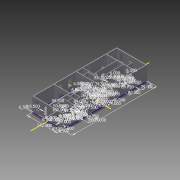
# Autodesk Inventor part: 2nd Floor
Saved by Autodesk Inventor 2013 SP2 (Build 170200200, 200)
## iProperties
Created: 2013-06-25
Part Number: 2nd Floor
Material: Generic
Document SubType Name: Modeling
Designer: Joey
Density: 1 g/cm^3
Author: Joey
Autodesk Inventor part; units mm, degrees
ref_plane "YZ Plane" through (0, 0, 0) normal (1, 0, 0) x (0, 1, 0)
ref_plane "XZ Plane" through (0, 0, 0) normal (0, 1, 0) x (-1, 0, 0)
ref_plane "XY Plane" through (0, 0, 0) normal (0, 0, 1) x (1, 0, 0)
sketch "Sketch1" plane through (0, 0, 0) normal (0, 1, 0) x (-1, 0, 0)
  line L0 (4302.76, 0) -> (-4302.76, 0) projected
  line L1 (0, -12001.5) -> (0, 12001.5) projected
  line L2 (3073.4, -8572.5) -> (-3073.4, -8572.5)
  line L3 (-3073.4, -8572.5) -> (-3073.4, 8572.5)
  line L4 (-3073.4, 8572.5) -> (3073.4, 8572.5)
  line L5 (3073.4, 8572.5) -> (3073.4, -8572.5)
  line L6 (2908.3, -8407.4) -> (-2908.3, -8407.4)
  line L7 (-2908.3, -8407.4) -> (-2908.3, 8407.4)
  line L8 (-2908.3, 5803.9) -> (-2908.3, 5918.2)
  line L9 (-2908.3, 8407.4) -> (-279.4, 8407.4)
  line L10 (-482.6, 8407.4) -> (2908.3, 8407.4)
  line L11 (2908.3, 8407.4) -> (2908.3, 4159.25)
  line L12 (2908.3, 4044.95) -> (2908.3, -8407.4)
  line L13 (-774.7, -292.1) -> (-774.7, -139.7)
  line L14 (2908.3, -139.7) -> (2908.3, -292.1)
  line L15 (961.4159, -292.1) -> (876.3, -292.1)
  line L16 (-514.35, -1485.9) -> (1289.2959, -1485.9)
  line L17 (2908.3, -1485.9) -> (2908.3, -1600.2)
  line L18 (806.45, -1600.2) -> (692.15, -1600.2)
  line L19 (692.15, -6248.4) -> (806.45, -6248.4)
  line L20 (692.15, -6248.4) -> (2908.3, -6248.4)
  line L21 (2908.3, -6248.4) -> (2908.3, -6400.8)
  line L22 (2908.3, -6400.8) -> (692.15, -6400.8)
  line L23 (692.15, -6400.8) -> (692.15, -6248.4)
  line L24 (-279.4, 4876.8) -> (-1993.9, 4876.8)
  line L25 (-2908.3, 4508.5) -> (-2908.3, 4394.2)
  line L26 (-2908.3, 2717.8) -> (-774.7, 2717.8)
  line L27 (-774.7, 2717.8) -> (-774.7, 2832.1)
  line L28 (-774.7, 2832.1) -> (-2908.3, 2832.1)
  line L29 (-2908.3, 2832.1) -> (-2908.3, 2717.8)
  line L30 (-774.7, -292.1) -> (-660.4, -292.1)
  line L31 (-2908.3, -1104.9) -> (-1504.95, -1104.9)
  line L32 (-1504.95, -1104.9) -> (-1504.95, -990.6)
  line L33 (-1504.95, -990.6) -> (-2908.3, -990.6)
  line L34 (-2908.3, -990.6) -> (-2908.3, -1104.9)
  line L35 (-2908.3, -1714.5) -> (-1504.95, -1714.5)
  line L36 (-1504.95, -1714.5) -> (-1504.95, -1600.2)
  line L37 (-1504.95, -1600.2) -> (-2908.3, -1600.2)
  line L38 (-2908.3, -1600.2) -> (-2908.3, -1714.5)
  line L39 (-2908.3, -139.7) -> (-2908.3, -292.1)
  line L40 (-774.7, -292.1) -> (-774.7, -139.7)
  line L41 (-514.35, -2616.2) -> (-514.35, -2730.5)
  line L42 (-2908.3, -2730.5) -> (-2908.3, -2616.2)
  line L43 (-514.35, -2616.2) -> (-628.65, -2616.2)
  line L44 (-628.65, -2616.2) -> (-628.65, -4235.45)
  line L45 (-628.65, -4235.45) -> (-514.35, -4235.45)
  line L46 (-514.35, -4235.45) -> (-514.35, -2616.2)
  line L47 (-514.35, -4235.45) -> (-2908.3, -4235.45)
  line L48 (-2908.3, -4235.45) -> (-2908.3, -4349.75)
  line L49 (-2908.3, -4349.75) -> (-514.35, -4349.75)
  line L50 (-514.35, -4349.75) -> (-514.35, -4235.45)
  line L51 (-514.35, -4349.75) -> (-628.65, -4349.75)
  line L52 (-628.65, -6248.4) -> (-514.35, -6248.4)
  line L53 (-514.35, -6248.4) -> (-2908.3, -6248.4)
  line L54 (-2908.3, -6248.4) -> (-2908.3, -6400.8)
  line L55 (-2908.3, -6400.8) -> (-514.35, -6400.8)
  line L56 (-514.35, -6400.8) -> (-514.35, -6248.4)
  line L57 (1670.05, -1600.2) -> (1555.75, -1600.2)
  line L58 (1555.75, -1600.2) -> (1555.75, -292.1)
  line L59 (1555.75, -292.1) -> (1670.05, -292.1)
  line L60 (1670.05, -292.1) -> (1670.05, -1600.2)
  line L61 (-2813.05, 5918.2) -> (-2908.3, 5918.2)
  line L62 (-2908.3, 8407.4) -> (-2813.05, 8407.4)
  line L63 (-660.4, 4762.5) -> (-774.7, 4762.5)
  line L64 (-774.7, 4762.5) -> (-774.7, 3625.85)
  line L65 (-774.7, 3625.85) -> (-660.4, 3625.85)
  line L66 (-660.4, 3625.85) -> (-660.4, 4762.5)
  line L67 (-514.35, -1485.9) -> (-514.35, -1600.2)
  line L68 (-1504.95, -292.1) -> (-1390.65, -292.1)
  line L69 (-1390.65, -292.1) -> (-1390.65, -2616.2)
  line L70 (-1390.65, -2616.2) -> (-1504.95, -2616.2)
  line L71 (-1504.95, -2616.2) -> (-1504.95, -292.1)
  line L72 (-2070.1, -292.1) -> (-1955.8, -292.1)
  line L73 (-1955.8, -292.1) -> (-1955.8, -1600.2)
  line L74 (-1955.8, -1600.2) -> (-2070.1, -1600.2)
  line L75 (-2070.1, -1600.2) -> (-2070.1, -292.1)
  line L76 (1555.75, -1320.8) -> (-514.35, -1320.8)
  line L77 (-514.35, -1320.8) -> (-514.35, -1206.5)
  line L78 (-514.35, -1206.5) -> (1555.75, -1206.5)
  line L79 (1555.75, -1206.5) -> (1555.75, -1320.8)
  line L80 (-514.35, -1206.5) -> (-400.05, -1206.5)
  line L81 (-400.05, -1206.5) -> (-400.05, -1600.2)
  line L82 (-400.05, -1600.2) -> (-514.35, -1600.2)
  line L83 (-514.35, -1600.2) -> (-514.35, -1206.5)
  line L84 (196.85, -139.7) -> (196.85, -292.1)
  line L85 (876.3, -139.7) -> (876.3, -292.1)
  line L86 (-2527.3, 8407.4) -> (-2413, 8407.4)
  line L87 (-2413, 8407.4) -> (-2413, 5918.2)
  line L88 (-2413, 5918.2) -> (-2527.3, 5918.2)
  line L89 (-2527.3, 5918.2) -> (-2527.3, 8407.4)
  line L90 (-774.7, -139.7) -> (196.85, -139.7)
  line L91 (876.3, -139.7) -> (2908.3, -139.7)
  line L92 (2908.3, -292.1) -> (876.3, -292.1)
  line L93 (196.85, -292.1) -> (-774.7, -292.1)
  line L94 (-514.35, -6248.4) -> (-311.15, -6248.4)
  line L95 (-311.15, -6248.4) -> (-311.15, -6400.8)
  line L96 (-311.15, -6400.8) -> (-514.35, -6400.8)
  line L97 (-514.35, -6400.8) -> (-514.35, -6248.4)
  line L98 (692.15, -6248.4) -> (488.95, -6248.4)
  line L99 (488.95, -6248.4) -> (488.95, -6400.8)
  line L100 (488.95, -6400.8) -> (692.15, -6400.8)
  line L101 (692.15, -6400.8) -> (692.15, -6248.4)
  line L102 (-774.7, -6400.8) -> (-660.4, -6400.8)
  line L103 (-1593.85, 5918.2) -> (-1657.35, 5918.2)
  line L104 (-1993.9, 4762.5) -> (-1879.6, 4762.5)
  line L105 (-660.4, 2832.1) -> (-660.4, 2870.2)
  line L106 (-660.4, 2870.2) -> (-774.7, 2870.2)
  line L107 (-774.7, 2870.2) -> (-774.7, 2832.1)
  line L108 (2908.3, 4159.25) -> (2908.3, 4044.95)
  line L109 (-127, 3956.05) -> (-279.4, 3956.05)
  line L110 (-279.4, 8407.4) -> (-127, 8407.4)
  line L111 (-1993.9, 3841.75) -> (-1993.9, 3956.05)
  line L112 (-1993.9, 5918.2) -> (-1879.6, 5918.2)
  line L113 (-1879.6, 4762.5) -> (-1993.9, 4762.5)
  line L114 (234.95, -1600.2) -> (349.25, -1600.2)
  line L115 (349.25, -1600.2) -> (349.25, -1905)
  line L116 (349.25, -1905) -> (234.95, -1905)
  line L117 (234.95, -1905) -> (234.95, -1600.2)
  line L118 (234.95, -1790.7) -> (692.15, -1790.7)
  line L119 (692.15, -1790.7) -> (692.15, -1905)
  line L120 (692.15, -1905) -> (234.95, -1905)
  line L121 (234.95, -1905) -> (234.95, -1790.7)
  line L122 (-127, 3956.05) -> (-127, 3841.75)
  line L123 (-127, 4191) -> (749.3, 4191)
  line L124 (749.3, 4191) -> (749.3, 4343.4)
  line L125 (749.3, 4343.4) -> (-127, 4343.4)
  line L126 (-127, 4343.4) -> (-127, 4191)
  line L127 (2032, 4191) -> (2908.3, 4191)
  line L128 (2908.3, 4191) -> (2908.3, 4343.4)
  line L129 (2908.3, 4343.4) -> (2032, 4343.4)
  line L130 (2032, 4343.4) -> (2032, 4191)
  line L131 (-1993.9, 3841.75) -> (-1879.6, 3841.75)
  line L132 (-1879.6, 3841.75) -> (-1879.6, 4762.5)
  line L133 (-1879.6, 4762.5) -> (-1993.9, 4762.5)
  line L134 (-1993.9, 4762.5) -> (-1993.9, 3841.75)
  line L135 (-1879.6, 3841.75) -> (-1993.9, 3841.75)
  line L136 (-279.4, 5918.2) -> (-279.4, 5803.9)
  line L137 (-279.4, 4876.8) -> (-279.4, 4762.5)
  line L138 (-1993.9, 4762.5) -> (-1879.6, 4762.5)
  line L139 (-1993.9, 4762.5) -> (-279.4, 4762.5)
  line L140 (-1993.9, 4876.8) -> (-2908.3, 4876.8)
  line L141 (-1993.9, 4762.5) -> (-2908.3, 4762.5)
  line L142 (-1231.9, -6400.8) -> (-1117.6, -6400.8)
  line L143 (-1117.6, -6400.8) -> (-1117.6, -7442.2)
  line L144 (-1117.6, -7442.2) -> (-1231.9, -7442.2)
  line L145 (-1231.9, -7442.2) -> (-1231.9, -6400.8)
  line L146 (692.15, -6045.2) -> (806.45, -6045.2)
  line L147 (692.15, -5334) -> (806.45, -5334)
  line L148 (692.15, -6045.2) -> (692.15, -6248.4)
  line L149 (806.45, -6248.4) -> (806.45, -6045.2)
  line L150 (-628.65, -4425.95) -> (-514.35, -4425.95)
  line L151 (-628.65, -5226.05) -> (-514.35, -5226.05)
  line L152 (692.15, -2971.8) -> (806.45, -2971.8)
  line L153 (692.15, -3771.9) -> (806.45, -3771.9)
  line L154 (692.15, -1600.2) -> (692.15, -2971.8)
  line L155 (692.15, -3771.9) -> (692.15, -5334)
  line L156 (806.45, -5334) -> (806.45, -3771.9)
  line L157 (806.45, -2971.8) -> (806.45, -1600.2)
  line L158 (-1339.85, -2616.2) -> (-1339.85, -2730.5)
  line L159 (-730.25, -2616.2) -> (-730.25, -2730.5)
  line L160 (-1555.75, -2616.2) -> (-1555.75, -2730.5)
  line L161 (-2165.35, -2616.2) -> (-2165.35, -2730.5)
  line L162 (-2165.35, -2730.5) -> (-2908.3, -2730.5)
  line L163 (-2908.3, -2616.2) -> (-2165.35, -2616.2)
  line L164 (-1555.75, -2616.2) -> (-1339.85, -2616.2)
  line L165 (-730.25, -2616.2) -> (-514.35, -2616.2)
  line L166 (-514.35, -2730.5) -> (-730.25, -2730.5)
  line L167 (-1339.85, -2730.5) -> (-1555.75, -2730.5)
  line L168 (-774.7, 1492.25) -> (-660.4, 1492.25)
  line L169 (-774.7, 736.6) -> (-660.4, 736.6)
  line L170 (-660.4, -292.1) -> (-660.4, 736.6)
  line L171 (-660.4, 1492.25) -> (-660.4, 2832.1)
  line L172 (-774.7, 2832.1) -> (-774.7, 1492.25)
  line L173 (-774.7, 736.6) -> (-774.7, -292.1)
  line L174 (-279.4, 8242.3) -> (-127, 8242.3)
  line L175 (-279.4, 7442.2) -> (-127, 7442.2)
  line L176 (-1447.8, 5918.2) -> (-1333.5, 5918.2)
  line L177 (-1333.5, 5918.2) -> (-1333.5, 4762.5)
  line L178 (-1333.5, 4762.5) -> (-1447.8, 4762.5)
  line L179 (-1447.8, 4762.5) -> (-1447.8, 5918.2)
  line L180 (-1993.9, 3956.05) -> (-1631.95, 3956.05)
  line L181 (-1631.95, 3956.05) -> (-1631.95, 3841.75)
  line L182 (-1631.95, 3841.75) -> (-1993.9, 3841.75)
  line L183 (-1993.9, 3841.75) -> (-1993.9, 3956.05)
  line L184 (-127, 3841.75) -> (-1022.35, 3841.75)
  line L185 (-1022.35, 3841.75) -> (-1022.35, 3956.05)
  line L186 (-1022.35, 3956.05) -> (-127, 3956.05)
  line L187 (-127, 3956.05) -> (-127, 3841.75)
  line L188 (-1111.25, 5918.2) -> (-1111.25, 5803.9)
  line L189 (-501.65, 5918.2) -> (-501.65, 5803.9)
  line L190 (-2908.3, 5918.2) -> (-1111.25, 5918.2)
  line L191 (-501.65, 5918.2) -> (-279.4, 5918.2)
  line L192 (-279.4, 5803.9) -> (-501.65, 5803.9)
  line L193 (-1111.25, 5803.9) -> (-2908.3, 5803.9)
  line L194 (-127, 8407.4) -> (-127, 8242.3)
  line L195 (-127, 7442.2) -> (-127, 3956.05)
  line L196 (-279.4, 3956.05) -> (-279.4, 7442.2)
  line L197 (-279.4, 8242.3) -> (-279.4, 8407.4)
  line L198 (-2794, -139.7) -> (-2794, -292.1)
  line L199 (-2184.4, -139.7) -> (-2184.4, -292.1)
  line L200 (-774.7, -139.7) -> (-2184.4, -139.7)
  line L201 (-2794, -139.7) -> (-2908.3, -139.7)
  line L202 (-2908.3, -292.1) -> (-2794, -292.1)
  line L203 (-2184.4, -292.1) -> (-774.7, -292.1)
  line L204 (2806.7, -1485.9) -> (2806.7, -1600.2)
  line L205 (2051.05, -1600.2) -> (2051.05, -1485.9)
  line L206 (-628.65, -4349.75) -> (-628.65, -4425.95)
  line L207 (-628.65, -5226.05) -> (-628.65, -6248.4)
  line L208 (-514.35, -6248.4) -> (-514.35, -5226.05)
  line L209 (-514.35, -4425.95) -> (-514.35, -4349.75)
  line L210 (2908.3, -1600.2) -> (2806.7, -1600.2)
  line L211 (2051.05, -1600.2) -> (-514.35, -1600.2)
  line L212 (-514.35, -1485.9) -> (2051.05, -1485.9)
  line L213 (2806.7, -1485.9) -> (2908.3, -1485.9)
  line L214 (-1993.9, 4876.8) -> (-1993.9, 4762.5)
  line L215 (-1231.9, -7327.9) -> (-520.7, -7327.9)
  line L216 (-520.7, -7327.9) -> (-520.7, -7442.2)
  line L217 (-520.7, -7442.2) -> (-1231.9, -7442.2)
  line L218 (-1231.9, -7442.2) -> (-1231.9, -7327.9)
  line L219 (-774.7, 2870.2) -> (-660.4, 2870.2)
  line L220 (-660.4, 2870.2) -> (-660.4, 1492.25)
  line L221 (-660.4, 1492.25) -> (-774.7, 1492.25)
  line L222 (-774.7, 1492.25) -> (-774.7, 2870.2)
  line L223 (-2908.3, 2832.1) -> (-2908.3, 4762.5)
  line L224 (-2908.3, 4876.8) -> (-2908.3, 5803.9)
  line L225 (-2908.3, 5918.2) -> (-2527.3, 5918.2)
  line L226 (-2908.3, 5918.2) -> (-2908.3, 8407.4)
  line L227 (-2908.3, 8407.4) -> (-279.4, 8407.4)
  line L228 (2908.3, 8407.4) -> (2908.3, 4343.4)
  line L229 (2908.3, 4191) -> (2908.3, -139.7)
  line L230 (-2908.3, 4876.8) -> (-279.4, 4876.8)
  line L231 (-279.4, 4876.8) -> (-279.4, 4762.5)
  line L232 (-279.4, 4762.5) -> (-2908.3, 4762.5)
  line L233 (-2908.3, 4762.5) -> (-2908.3, 4876.8)
  line L234 (-2908.3, 8407.4) -> (2908.3, 8407.4)
  line L235 (2908.3, 8407.4) -> (2908.3, -8407.4)
  line L236 (2908.3, -8407.4) -> (-2908.3, -8407.4)
  line L237 (-2908.3, -8407.4) -> (-2908.3, 8407.4)
  point P0 (0, 0)
  point P1 (-2470.15, 8407.4)
  point P2 (-2908.3, 5861.05)
  point P3 (-2908.3, 2774.95)
  point P4 (-2908.3, -215.9)
  point P5 (-2908.3, -1047.75)
  point P6 (-2908.3, -1657.35)
  point P7 (-2908.3, -2673.35)
  point P8 (-2908.3, -4292.6)
  point P9 (-2908.3, -6324.6)
  point P10 (2908.3, -1543.05)
  point P11 (2908.3, -6324.6)
  point P12 (2908.3, -215.9)
  point P13 (-203.2, 8407.4)
  dimension "d0" = 17145
  dimension "d2" = 6146.8
  dimension "d14" = 165.1
  dimension "d15" = 165.1
  dimension "d22" = 152.4
  dimension "d25" = 114.3
  dimension "d30" = 114.3
  dimension "d36" = 114.3
  dimension "d38" = 114.3
  dimension "d42" = 152.4
  dimension "d44" = 114.3
  dimension "d45" = 165.1
  dimension "d54" = 114.3
  dimension "d64" = 165.1
  dimension "d66" = 165.1
  dimension "d67" = 2133.6
  dimension "d71" = 114.3
  dimension "d73" = 2946.4
  dimension "d74" = 114.3
  dimension "d80" = 876.3
  dimension "d81" = 1587.5
  dimension "d82" = 679.45
  dimension "d83" = 114.3
  dimension "d92" = 2032
  dimension "d93" = 152.4
  dimension "d95" = 914.4
  dimension "d96" = 152.4
  dimension "d99" = 203.2
  dimension "d100" = 203.2
  dimension "d112" = 38.1
  dimension "d113" = 755.65
  dimension "d117" = 838.2
  dimension "d128" = 914.4
  dimension "d133" = 114.3
  dimension "d134" = 114.3
  dimension "d137" = 152.4
  dimension "d138" = 1282.7
  dimension "d141" = 114.3
  dimension "d145" = 4064
  dimension "d146" = 876.3
  dimension "d147" = 1009.65
  dimension "d152" = 114.3
  dimension "d162" = 114.3
  dimension "d163" = 114.3
  dimension "d164" = 114.3
  dimension "d165" = 1930.4
  dimension "d166" = 2006.6
  dimension "d173" = 165.1
  dimension "d175" = 1016
  dimension "d176" = 609.6
  dimension "d177" = 114.3
  dimension "d178" = 1041.4
  dimension "d179" = 1676.4
  dimension "d180" = 203.2
  dimension "d181" = 711.2
  dimension "d184" = 114.3
  dimension "d187" = 76.2
  dimension "d188" = 800.1
  dimension "d189" = 2032
  dimension "d191" = 1066.8
  dimension "d192" = 800.1
  dimension "d193" = 1206.5
  dimension "d194" = 2101.85
  dimension "d195" = 457.2
  constraints: 470 end point, 126 parallel, 91 perpendicular, 54 horizontal, 47 collinear, 30 point on line, 13 midpoint, 4 vertical, 16 other
  measures "d0" distance between parallel lines of L4 L2
  measures "d2" distance between parallel lines of L3 L5
  measures "d14" distance between parallel lines of L4 L10
  measures "d15" distance between parallel lines of L4 L9
  measures "d22" distance between parallel lines of L20 L22
  measures "d25" distance between parallel lines of L28 L26
  measures "d30" distance between parallel lines of L37 L35
  measures "d36" distance between parallel lines of L46 L44
  measures "d38" distance between parallel lines of L47 L49
  measures "d42" distance between parallel lines of L53 L55
  measures "d44" distance between parallel lines of L60 L58
  measures "d45" distance between parallel lines of L5 L12
  measures "d54" distance between parallel lines of L66 L64
  measures "d64" distance between parallel lines of L5 L11
  measures "d66" distance between parallel lines of L2 L6
  measures "d71" distance between parallel lines of L75 L73
  measures "d73" distance between parallel lines of L58 L69
  measures "d74" distance between parallel lines of L76 L78
  measures "d80" distance between parallel lines of L69 L83
  measures "d81" distance between parallel lines of L69 L84
  measures "d82" distance between parallel lines of L84 L85
  measures "d83" distance between parallel lines of L89 L87
  measures "d92" distance between parallel lines of L12 L85
  measures "d93" distance between parallel lines of L92 L91
  measures "d95" distance between parallel lines of L78 L93
  measures "d96" distance between parallel lines of L93 L90
  measures "d99" distance between parallel lines of L97 L95
  measures "d100" distance between parallel lines of L101 L99
  measures "d112" distance between parallel lines of L28 L106
  measures "d113" distance between parallel lines of L106 L65
  measures "d133" distance between parallel lines of L120 L118
  measures "d134" distance between parallel lines of L117 L115
  measures "d137" distance between parallel lines of L123 L125
  measures "d138" distance between parallel lines of L130 L124
  measures "d141" distance between parallel lines of L134 L132
  measures "d145" distance between parallel lines of L129 L10
  measures "d146" distance from line of L12.start L130
  measures "d147" distance between parallel lines of L28 L131
  measures "d152" distance between parallel lines of L139 L24
  measures "d162" distance between parallel lines of L83 L81
  measures "d163" distance between parallel lines of L31 L33
  measures "d164" distance between parallel lines of L69 L71
  measures "d165" distance between parallel lines of L28 L139
  measures "d166" distance between parallel lines of L6 L55
  measures "d175" distance of point (-2908.3, -2673.35) point (-2908.3, -1657.35)
  measures "d176" distance of point (-2908.3, -1047.75) point (-2908.3, -1657.35)
  measures "d177" distance between parallel lines of L145 L143
  measures "d178" distance between parallel lines of L102 L144
  measures "d180" distance between parallel lines of L98 L146
  measures "d181" distance between parallel lines of L146 L147
  measures "d184" distance between parallel lines of L149 L148
  measures "d187" distance between parallel lines of L49 L150
  measures "d188" distance between parallel lines of L151 L150
  measures "d189" distance of point (-2908.3, -6324.6) point (-2908.3, -4292.6)
  measures "d191" distance between parallel lines of L120 L152
  measures "d192" distance between parallel lines of L152 L153
  measures "d193" distance between parallel lines of L46 L155
  measures "d194" distance between parallel lines of L12 L156
  measures "d195" distance between parallel lines of L154 L117
extrude "Extrusion1" add sketch "Sketch1" along normal blind 2844.8 contours L5 L2 L1 L6 L12 L0 | L0 L12 L108 L11 L10 L1 L4 L5 | L12 L92 L59 L15 L85 L91 | L1 L10 L9 L7 L0 L3 L4 | L2 L3 L0 L7 L6 L1 | L170 L90 L173 L0 | L0 L173 L169 L170 | L90 L84 L93 L1 | L1 L93 L170 L90 | L123 L126 L125 L1 | L1 L125 L124 L123 | L170 L30 L13 L90 | L195 L109 L196 L137 L136 L175 L126 | L127 L130 L129 L11 | L12 L210 L204 L213 | L60 L212 L58 L59 | L194 L174 L197 L10 | L211 L81 L16 L1 | L1 L16 L212 L58 L211 L18 L114 | L13 L203 L68 L72 L199 L200 | L78 L58 L76 L1 | L1 L76 L81 L78 | L122 L184 L66 L186 L109 | L212 L205 L211 L60 | L60 L57 L58 L212 | L114 L115 L118 L117 | L82 L67 L16 L81 | L22 L23 L19 L20 L12 | L7 L53 L52 L56 L55 | L201 L198 L202 L7 | L7 L28 L27 L26 | L81 L76 L77 L78 | L16 L83 L76 L81 | L211 L154 L118 L115 | L118 L115 L116 L117 | L100 L99 L98 L23 | L55 L143 L215 L145 | L27 L107 L106 L105 L171 L168 L172 | L69 L70 L71 L36 L32 L68 | L186 L64 L63 L66 | L66 L184 L64 L186 | L139 L63 L177 L24 L137 | L66 L65 L64 L184 | L19 L148 L146 L149 | L87 L88 L89 L9 | L118 L119 L120 L115 | L18 L157 L152 L154 L119 | L7 L47 L45 L50 L49 | L207 L151 L208 L52 | L215 L143 L144 L145 | L33 L75 L31 L7 | L164 L158 L167 L160 L70 | L72 L73 L33 L75 | L136 L192 L189 L191 | L64 L184 L185 L186 | L190 L112 L103 L179 L193 L7 L61 L88 | L49 L209 L150 L206 | L94 L95 L96 L56 | L215 L216 L217 L143 | L33 L73 L31 L75 | L32 L31 L73 L33 | L177 L139 L179 L24 | L24 L179 L193 L177 | L7 L163 L161 L162 | L44 L166 L46 L45 | L37 L36 L35 L7 | L31 L73 L37 L75 | L7 L140 L214 L141 | L179 L139 L104 L214 L24 | L193 L179 L176 L177 | L177 L190 L188 L193 | L166 L159 L165 L44 | L44 L43 L41 L166 | L104 L132 L180 L134 | L180 L132 L131 L111 | L180 L181 L182 L132 | L155 L153 L156 L147
extrude "Extrusion2" add sketch "Sketch1" along normal blind 2844.8 contours L118 L115 L116 L117 | L118 L119 L120 L115
extrude "Extrusion3" cut sketch "Sketch1" along normal blind 2844.8 contours L211 L154 L118 L115
sketch "Sketch2" plane through (0, 0, 0) normal (0, -1, 0) x (1, 0, 0)
  line L0 (1993.9, 3841.75) -> (1631.95, 3841.75) projected
  line L1 (1993.9, 4762.5) -> (1993.9, 3841.75) projected
  line L2 (1231.9, -7442.2) -> (520.7, -7442.2) projected
  line L3 (1231.9, -6400.8) -> (1231.9, -7442.2) projected
  line L4 (-3073.4, 8572.5) -> (3073.4, 8572.5)
  line L5 (3073.4, 8572.5) -> (3073.4, -8572.5)
  line L6 (3073.4, -8572.5) -> (-3073.4, -8572.5)
  line L7 (-3073.4, -8572.5) -> (-3073.4, 8572.5)
  line L8 (520.7, -7442.2) -> (2908.3, -7442.2)
  line L9 (2908.3, -7442.2) -> (2908.3, -8407.4)
  line L10 (2908.3, -8407.4) -> (520.7, -8407.4)
  line L11 (520.7, -8407.4) -> (520.7, -7442.2)
  line L12 (2908.3, -8407.4) -> (1231.9, -8407.4)
  line L13 (1231.9, -8407.4) -> (1231.9, -6400.8)
  line L14 (1231.9, -6400.8) -> (2908.3, -6400.8)
  line L15 (2908.3, -6400.8) -> (2908.3, -8407.4)
  line L16 (1739.9, 3841.75) -> (2908.3, 3841.75)
  line L17 (2908.3, 3841.75) -> (2908.3, 2832.1)
  line L18 (2908.3, 2832.1) -> (1739.9, 2832.1)
  line L19 (1739.9, 2832.1) -> (1739.9, 3841.75)
  line L20 (1993.9, 4762.5) -> (2908.3, 4762.5)
  line L21 (2908.3, 4762.5) -> (2908.3, 2832.1)
  line L22 (2908.3, 2832.1) -> (1993.9, 2832.1)
  line L23 (1993.9, 2832.1) -> (1993.9, 4762.5)
  point P0 (0, 0)
  dimension "d242" = 1168.4
  constraints: 40 end point, 10 parallel, 5 horizontal, 5 perpendicular, 1 point on line
  measures "d242" distance between parallel lines of L17 L19
extrude "Extrusion4" add sketch "Sketch2" along normal blind 463.55
sketch "Sketch3" plane through (0, 2844.8, 0) normal (0, 1, 0) x (1, 0, 0)
  line L0 (-692.15, 1790.7) -> (-349.25, 1790.7) projected
  line L1 (-349.25, 1790.7) -> (-349.25, 1600.2) projected
  line L2 (-349.25, 1600.2) -> (-692.15, 1600.2) projected
  line L3 (-692.15, 1600.2) -> (-692.15, 1790.7) projected
  line L4 (-876.3, 139.7) -> (-2908.3, 139.7) projected
  line L5 (-876.3, 292.1) -> (-876.3, 139.7) projected
  line L6 (-1555.75, 292.1) -> (-876.3, 292.1) projected
  line L7 (-1555.75, 1206.5) -> (-1555.75, 292.1) projected
  line L8 (514.35, 1206.5) -> (-1555.75, 1206.5) projected
  line L9 (514.35, 1600.2) -> (514.35, 1206.5) projected
  line L10 (-234.95, 1600.2) -> (514.35, 1600.2) projected
  line L11 (-234.95, 1600.2) -> (-234.95, 1905) projected
  line L12 (-234.95, 1905) -> (-692.15, 1905) projected
  line L13 (-692.15, 2971.8) -> (-692.15, 1905) projected
  line L14 (-806.45, 6248.4) -> (-2908.3, 6248.4) projected
  line L15 (1390.65, 292.1) -> (1390.65, 2616.2) projected
  line L16 (400.05, 1320.8) -> (400.05, 1485.9) projected
  line L17 (-1555.75, 1320.8) -> (400.05, 1320.8) projected
  line L18 (-1555.75, 1485.9) -> (-1555.75, 1320.8) projected
  line L19 (400.05, 1485.9) -> (-1555.75, 1485.9) projected
  line L20 (-692.15, 5334) -> (-692.15, 3771.9) projected
  line L21 (-806.45, 5334) -> (-692.15, 5334) projected
  line L22 (-806.45, 3771.9) -> (-806.45, 5334) projected
  line L23 (-692.15, 3771.9) -> (-806.45, 3771.9) projected
  line L24 (-1555.75, 292.1) -> (1390.65, 292.1)
  line L25 (1390.65, 292.1) -> (1390.65, 1600.2)
  line L26 (1390.65, 1600.2) -> (-1555.75, 1600.2)
  line L27 (-1555.75, 1600.2) -> (-1555.75, 292.1)
  line L28 (1390.65, 1600.2) -> (-692.15, 1600.2)
  line L29 (-692.15, 1600.2) -> (-692.15, 2616.2)
  line L30 (-692.15, 2616.2) -> (1390.65, 2616.2)
  line L31 (1390.65, 2616.2) -> (1390.65, 1600.2)
  line L32 (-692.15, 2616.2) -> (514.35, 2616.2)
  line L33 (514.35, 2616.2) -> (514.35, 6248.4)
  line L34 (514.35, 6248.4) -> (-692.15, 6248.4)
  line L35 (-692.15, 6248.4) -> (-692.15, 2616.2)
  line L36 (660.4, -4762.5) -> (-2908.3, -4762.5)
  line L37 (-2908.3, -4762.5) -> (-2908.3, 292.1)
  line L38 (-2908.3, 292.1) -> (660.4, 292.1)
  line L39 (660.4, 292.1) -> (660.4, -4762.5)
  line L40 (-2908.3, 292.1) -> (-1555.75, 292.1)
  line L41 (-1555.75, 292.1) -> (-1555.75, 6248.4)
  line L42 (-1555.75, 6248.4) -> (-2908.3, 6248.4)
  line L43 (-2908.3, 6248.4) -> (-2908.3, 292.1)
  line L44 (-692.15, 1600.2) -> (-1555.75, 1600.2)
  line L45 (-1555.75, 1600.2) -> (-1555.75, 6248.4)
  line L46 (-1555.75, 6248.4) -> (-692.15, 6248.4)
  line L47 (-692.15, 6248.4) -> (-692.15, 1600.2)
  line L48 (514.35, 2616.2) -> (2908.3, 2616.2)
  line L49 (2908.3, 2616.2) -> (2908.3, 8407.4)
  line L50 (2908.3, 8407.4) -> (514.35, 8407.4)
  line L51 (514.35, 8407.4) -> (514.35, 2616.2)
  line L52 (2908.3, 8407.4) -> (-2908.3, 8407.4)
  line L53 (-2908.3, 8407.4) -> (-2908.3, 6248.4)
  line L54 (-2908.3, 6248.4) -> (2908.3, 6248.4)
  line L55 (2908.3, 6248.4) -> (2908.3, 8407.4)
  line L56 (-2908.3, -8407.4) -> (2908.3, -8407.4)
  line L57 (2908.3, -8407.4) -> (2908.3, -4762.5)
  line L58 (2908.3, -4762.5) -> (-2908.3, -4762.5)
  line L59 (-2908.3, -4762.5) -> (-2908.3, -8407.4)
  line L60 (-2908.3, -4191) -> (-2603.5, -4191)
  line L61 (-2603.5, -4191) -> (-2603.5, 139.7)
  line L62 (-2603.5, 139.7) -> (-2908.3, 139.7)
  line L63 (-2908.3, 139.7) -> (-2908.3, -4191)
  line L64 (-2908.3, -4762.5) -> (660.4, -4762.5)
  line L65 (660.4, -4762.5) -> (660.4, -4191)
  line L66 (660.4, -4191) -> (-2908.3, -4191)
  line L67 (-2908.3, -4191) -> (-2908.3, -4762.5)
  line L68 (660.4, -4191) -> (-2603.5, -4191)
  line L69 (-2603.5, -4191) -> (-2603.5, 0)
  line L70 (-2603.5, 0) -> (660.4, 0)
  line L71 (660.4, 0) -> (660.4, -4191)
  line L72 (774.7, -2717.8) -> (2908.3, -2717.8) projected
  line L73 (774.7, -2717.8) -> (2908.3, -2717.8)
  line L74 (2908.3, -2717.8) -> (2908.3, 292.1)
  line L75 (2908.3, 292.1) -> (774.7, 292.1)
  line L76 (774.7, 292.1) -> (774.7, -2717.8)
  line L77 (2908.3, 292.1) -> (1390.65, 292.1)
  line L78 (1390.65, 292.1) -> (1390.65, 2616.2)
  line L79 (1390.65, 2616.2) -> (2908.3, 2616.2)
  line L80 (2908.3, 2616.2) -> (2908.3, 292.1)
  line L81 (-692.15, 5334) -> (-806.45, 5334) projected
  line L82 (-692.15, 3771.9) -> (-692.15, 5334) projected
  line L83 (-806.45, 3771.9) -> (-692.15, 3771.9) projected
  line L84 (-806.45, 5334) -> (-806.45, 3771.9) projected
  line L85 (520.7, 7442.2) -> (520.7, 7327.9) projected
  line L86 (520.7, 7442.2) -> (520.7, 8407.4) projected
  line L87 (520.7, 8407.4) -> (-2908.3, 8407.4) projected
  line L88 (-2908.3, 8407.4) -> (-2908.3, 6400.8) projected
  line L89 (-488.95, 6400.8) -> (-2908.3, 6400.8) projected
  line L90 (-488.95, 6248.4) -> (-488.95, 6400.8) projected
  line L91 (-692.15, 6248.4) -> (-488.95, 6248.4) projected
  line L92 (-692.15, 6045.2) -> (-692.15, 6248.4) projected
  line L93 (-806.45, 6045.2) -> (-692.15, 6045.2) projected
  line L94 (-806.45, 6248.4) -> (-806.45, 6045.2) projected
  line L95 (-2908.3, 6248.4) -> (-806.45, 6248.4) projected
  line L96 (-2908.3, 6248.4) -> (-2908.3, 1600.2) projected
  line L97 (-2806.7, 1600.2) -> (-2908.3, 1600.2) projected
  line L98 (-2806.7, 1485.9) -> (-2806.7, 1600.2) projected
  line L99 (-2908.3, 1485.9) -> (-2806.7, 1485.9) projected
  line L100 (-2908.3, 1485.9) -> (-2908.3, 292.1) projected
  line L101 (-1670.05, 292.1) -> (-2908.3, 292.1) projected
  line L102 (-1670.05, 1485.9) -> (-1670.05, 292.1) projected
  line L103 (-2051.05, 1485.9) -> (-1670.05, 1485.9) projected
  line L104 (-2051.05, 1600.2) -> (-2051.05, 1485.9) projected
  line L105 (-806.45, 1600.2) -> (-2051.05, 1600.2) projected
  line L106 (-806.45, 2971.8) -> (-806.45, 1600.2) projected
  line L107 (-692.15, 2971.8) -> (-806.45, 2971.8) projected
  line L108 (-692.15, 1905) -> (-692.15, 2971.8) projected
  line L109 (-234.95, 1905) -> (-692.15, 1905) projected
  line L110 (-234.95, 1600.2) -> (-234.95, 1905) projected
  line L111 (514.35, 1600.2) -> (-234.95, 1600.2) projected
  line L112 (514.35, 1206.5) -> (514.35, 1600.2) projected
  line L113 (-1555.75, 1206.5) -> (514.35, 1206.5) projected
  line L114 (-1555.75, 292.1) -> (-1555.75, 1206.5) projected
  line L115 (-876.3, 292.1) -> (-1555.75, 292.1) projected
  line L116 (-876.3, 139.7) -> (-876.3, 292.1) projected
  line L117 (-2908.3, 139.7) -> (-876.3, 139.7) projected
  line L118 (-2908.3, 139.7) -> (-2908.3, -4191) projected
  line L119 (-2032, -4191) -> (-2908.3, -4191) projected
  line L120 (-2032, -4343.4) -> (-2032, -4191) projected
  line L121 (-2908.3, -4343.4) -> (-2032, -4343.4) projected
  line L122 (-2908.3, -4343.4) -> (-2908.3, -8407.4) projected
  line L123 (-2908.3, -8407.4) -> (127, -8407.4) projected
  line L124 (127, -8242.3) -> (127, -8407.4) projected
  line L125 (279.4, -8242.3) -> (127, -8242.3) projected
  line L126 (279.4, -8407.4) -> (279.4, -8242.3) projected
  line L127 (279.4, -8407.4) -> (2413, -8407.4) projected
  line L128 (2413, -5918.2) -> (2413, -8407.4) projected
  line L129 (1111.25, -5918.2) -> (2413, -5918.2) projected
  line L130 (1111.25, -5803.9) -> (1111.25, -5918.2) projected
  line L131 (1333.5, -5803.9) -> (1111.25, -5803.9) projected
  line L132 (1333.5, -4876.8) -> (1333.5, -5803.9) projected
  line L133 (279.4, -4876.8) -> (1333.5, -4876.8) projected
  line L134 (279.4, -5803.9) -> (279.4, -4876.8) projected
  line L135 (501.65, -5803.9) -> (279.4, -5803.9) projected
  line L136 (501.65, -5918.2) -> (501.65, -5803.9) projected
  line L137 (279.4, -5918.2) -> (501.65, -5918.2) projected
  line L138 (279.4, -7442.2) -> (279.4, -5918.2) projected
  line L139 (127, -7442.2) -> (279.4, -7442.2) projected
  line L140 (127, -4343.4) -> (127, -7442.2) projected
  line L141 (-749.3, -4343.4) -> (127, -4343.4) projected
  line L142 (-749.3, -4191) -> (-749.3, -4343.4) projected
  line L143 (127, -4191) -> (-749.3, -4191) projected
  line L144 (127, -3841.75) -> (127, -4191) projected
  line L145 (660.4, -3841.75) -> (127, -3841.75) projected
  line L146 (660.4, -3625.85) -> (660.4, -3841.75) projected
  line L147 (774.7, -3625.85) -> (660.4, -3625.85) projected
  line L148 (774.7, -3841.75) -> (774.7, -3625.85) projected
  line L149 (1022.35, -3841.75) -> (774.7, -3841.75) projected
  line L150 (1022.35, -3956.05) -> (1022.35, -3841.75) projected
  line L151 (774.7, -3956.05) -> (1022.35, -3956.05) projected
  line L152 (774.7, -4762.5) -> (774.7, -3956.05) projected
  line L153 (1879.6, -4762.5) -> (774.7, -4762.5) projected
  line L154 (1879.6, -3956.05) -> (1879.6, -4762.5) projected
  line L155 (1631.95, -3956.05) -> (1879.6, -3956.05) projected
  line L156 (1631.95, -3841.75) -> (1631.95, -3956.05) projected
  line L157 (1739.9, -3841.75) -> (1631.95, -3841.75) projected
  line L158 (1739.9, -3841.75) -> (1739.9, -2832.1) projected
  line L159 (774.7, -2832.1) -> (1739.9, -2832.1) projected
  line L160 (774.7, -2870.2) -> (774.7, -2832.1) projected
  line L161 (660.4, -2870.2) -> (774.7, -2870.2) projected
  line L162 (660.4, -1492.25) -> (660.4, -2870.2) projected
  line L163 (774.7, -1492.25) -> (660.4, -1492.25) projected
  line L164 (774.7, -2717.8) -> (774.7, -1492.25) projected
  line L165 (2908.3, -2717.8) -> (774.7, -2717.8) projected
  line L166 (2908.3, -2717.8) -> (2908.3, 139.7) projected
  line L167 (2794, 139.7) -> (2908.3, 139.7) projected
  line L168 (2794, 292.1) -> (2794, 139.7) projected
  line L169 (2908.3, 292.1) -> (2794, 292.1) projected
  line L170 (2908.3, 292.1) -> (2908.3, 990.6) projected
  line L171 (2070.1, 990.6) -> (2908.3, 990.6) projected
  line L172 (2070.1, 292.1) -> (2070.1, 990.6) projected
  line L173 (2184.4, 292.1) -> (2070.1, 292.1) projected
  line L174 (2184.4, 139.7) -> (2184.4, 292.1) projected
  line L175 (774.7, 139.7) -> (2184.4, 139.7) projected
  line L176 (774.7, -736.6) -> (774.7, 139.7) projected
  line L177 (660.4, -736.6) -> (774.7, -736.6) projected
  line L178 (660.4, 139.7) -> (660.4, -736.6) projected
  line L179 (-196.85, 139.7) -> (660.4, 139.7) projected
  line L180 (-196.85, 292.1) -> (-196.85, 139.7) projected
  line L181 (1390.65, 292.1) -> (-196.85, 292.1) projected
  line L182 (1390.65, 2616.2) -> (1390.65, 292.1) projected
  line L183 (1339.85, 2616.2) -> (1390.65, 2616.2) projected
  line L184 (1339.85, 2730.5) -> (1339.85, 2616.2) projected
  line L185 (1555.75, 2730.5) -> (1339.85, 2730.5) projected
  line L186 (1555.75, 2616.2) -> (1555.75, 2730.5) projected
  line L187 (1504.95, 2616.2) -> (1555.75, 2616.2) projected
  line L188 (1504.95, 1714.5) -> (1504.95, 2616.2) projected
  line L189 (2908.3, 1714.5) -> (1504.95, 1714.5) projected
  line L190 (2908.3, 1714.5) -> (2908.3, 2616.2) projected
  line L191 (2165.35, 2616.2) -> (2908.3, 2616.2) projected
  line L192 (2165.35, 2730.5) -> (2165.35, 2616.2) projected
  line L193 (2908.3, 2730.5) -> (2165.35, 2730.5) projected
  line L194 (2908.3, 2730.5) -> (2908.3, 4235.45) projected
  line L195 (628.65, 4235.45) -> (2908.3, 4235.45) projected
  line L196 (628.65, 2730.5) -> (628.65, 4235.45) projected
  line L197 (730.25, 2730.5) -> (628.65, 2730.5) projected
  line L198 (730.25, 2616.2) -> (730.25, 2730.5) projected
  line L199 (514.35, 2616.2) -> (730.25, 2616.2) projected
  line L200 (514.35, 4425.95) -> (514.35, 2616.2) projected
  line L201 (628.65, 4425.95) -> (514.35, 4425.95) projected
  line L202 (628.65, 4349.75) -> (628.65, 4425.95) projected
  line L203 (2908.3, 4349.75) -> (628.65, 4349.75) projected
  line L204 (2908.3, 4349.75) -> (2908.3, 6248.4) projected
  line L205 (628.65, 6248.4) -> (2908.3, 6248.4) projected
  line L206 (628.65, 5226.05) -> (628.65, 6248.4) projected
  line L207 (514.35, 5226.05) -> (628.65, 5226.05) projected
  line L208 (514.35, 6248.4) -> (514.35, 5226.05) projected
  line L209 (311.15, 6248.4) -> (514.35, 6248.4) projected
  line L210 (311.15, 6400.8) -> (311.15, 6248.4) projected
  line L211 (1117.6, 6400.8) -> (311.15, 6400.8) projected
  line L212 (1117.6, 7327.9) -> (1117.6, 6400.8) projected
  line L213 (520.7, 7327.9) -> (1117.6, 7327.9) projected
  line L214 (774.7, -3956.05) -> (1879.6, -3956.05)
  line L215 (1879.6, -3956.05) -> (1879.6, -4762.5)
  line L216 (1879.6, -4762.5) -> (774.7, -4762.5)
  line L217 (774.7, -4762.5) -> (774.7, -3956.05)
  line L218 (-488.95, 6400.8) -> (311.15, 6400.8)
  line L219 (311.15, 6400.8) -> (311.15, 6248.4)
  line L220 (311.15, 6248.4) -> (-488.95, 6248.4)
  line L221 (-488.95, 6248.4) -> (-488.95, 6400.8)
  line L222 (-806.45, 6045.2) -> (-692.15, 6045.2)
  line L223 (-692.15, 6045.2) -> (-692.15, 5334)
  line L224 (-692.15, 5334) -> (-806.45, 5334)
  line L225 (-806.45, 5334) -> (-806.45, 6045.2)
  line L226 (514.35, 5226.05) -> (628.65, 5226.05)
  line L227 (628.65, 5226.05) -> (628.65, 4425.95)
  line L228 (628.65, 4425.95) -> (514.35, 4425.95)
  line L229 (514.35, 4425.95) -> (514.35, 5226.05)
  line L230 (-806.45, 3771.9) -> (-692.15, 3771.9)
  line L231 (-692.15, 3771.9) -> (-692.15, 2971.8)
  line L232 (-692.15, 2971.8) -> (-806.45, 2971.8)
  line L233 (-806.45, 2971.8) -> (-806.45, 3771.9)
  line L234 (730.25, 2730.5) -> (1339.85, 2730.5)
  line L235 (1339.85, 2730.5) -> (1339.85, 2616.2)
  line L236 (1339.85, 2616.2) -> (730.25, 2616.2)
  line L237 (730.25, 2616.2) -> (730.25, 2730.5)
  line L238 (1555.75, 2730.5) -> (2165.35, 2730.5)
  line L239 (2165.35, 2730.5) -> (2165.35, 2616.2)
  line L240 (2165.35, 2616.2) -> (1555.75, 2616.2)
  line L241 (1555.75, 2616.2) -> (1555.75, 2730.5)
  line L242 (2184.4, 292.1) -> (2794, 292.1)
  line L243 (2794, 292.1) -> (2794, 139.7)
  line L244 (2794, 139.7) -> (2184.4, 139.7)
  line L245 (2184.4, 139.7) -> (2184.4, 292.1)
  line L246 (1504.95, 990.6) -> (1955.8, 990.6) projected
  line L247 (1504.95, 292.1) -> (1504.95, 990.6) projected
  line L248 (1955.8, 292.1) -> (1504.95, 292.1) projected
  line L249 (1955.8, 990.6) -> (1955.8, 292.1) projected
  line L250 (1955.8, 1104.9) -> (1504.95, 1104.9) projected
  line L251 (1955.8, 1600.2) -> (1955.8, 1104.9) projected
  line L252 (1504.95, 1600.2) -> (1955.8, 1600.2) projected
  line L253 (1504.95, 1104.9) -> (1504.95, 1600.2) projected
  line L254 (2908.3, 1104.9) -> (2070.1, 1104.9) projected
  line L255 (2908.3, 1104.9) -> (2908.3, 1600.2) projected
  line L256 (2070.1, 1600.2) -> (2908.3, 1600.2) projected
  line L257 (2070.1, 1104.9) -> (2070.1, 1600.2) projected
  line L258 (660.4, -736.6) -> (774.7, -736.6)
  line L259 (774.7, -736.6) -> (774.7, -1492.25)
  line L260 (774.7, -1492.25) -> (660.4, -1492.25)
  line L261 (660.4, -1492.25) -> (660.4, -736.6)
  line L262 (660.4, -2870.2) -> (774.7, -2870.2)
  line L263 (774.7, -2870.2) -> (774.7, -3625.85)
  line L264 (774.7, -3625.85) -> (660.4, -3625.85)
  line L265 (660.4, -3625.85) -> (660.4, -2870.2)
  line L266 (1022.35, -3841.75) -> (1631.95, -3841.75)
  line L267 (1631.95, -3841.75) -> (1631.95, -3956.05)
  line L268 (1631.95, -3956.05) -> (1022.35, -3956.05)
  line L269 (1022.35, -3956.05) -> (1022.35, -3841.75)
  line L270 (-2032, -4191) -> (-749.3, -4191)
  line L271 (-749.3, -4191) -> (-749.3, -4343.4)
  line L272 (-749.3, -4343.4) -> (-2032, -4343.4)
  line L273 (-2032, -4343.4) -> (-2032, -4191)
  line L274 (-876.3, 139.7) -> (-196.85, 139.7)
  line L275 (-196.85, 139.7) -> (-196.85, 292.1)
  line L276 (-196.85, 292.1) -> (-876.3, 292.1)
  line L277 (-876.3, 292.1) -> (-876.3, 139.7)
  line L278 (514.35, 1206.5) -> (1390.65, 1206.5)
  line L279 (1390.65, 1206.5) -> (1390.65, 1358.9)
  line L280 (1390.65, 1358.9) -> (514.35, 1358.9)
  line L281 (514.35, 1358.9) -> (514.35, 1206.5)
  line L282 (-2806.7, 1600.2) -> (-2051.05, 1600.2)
  line L283 (-2051.05, 1600.2) -> (-2051.05, 1485.9)
  line L284 (-2051.05, 1485.9) -> (-2806.7, 1485.9)
  line L285 (-2806.7, 1485.9) -> (-2806.7, 1600.2)
  line L286 (501.65, -5803.9) -> (1111.25, -5803.9)
  line L287 (1111.25, -5803.9) -> (1111.25, -5918.2)
  line L288 (1111.25, -5918.2) -> (501.65, -5918.2)
  line L289 (501.65, -5918.2) -> (501.65, -5803.9)
  line L290 (127, -7442.2) -> (279.4, -7442.2)
  line L291 (279.4, -7442.2) -> (279.4, -8242.3)
  line L292 (279.4, -8242.3) -> (127, -8242.3)
  line L293 (127, -8242.3) -> (127, -7442.2)
  line L294 (1111.25, -5918.2) -> (1111.25, -5803.9) projected
  line L295 (2413, -5918.2) -> (1111.25, -5918.2) projected
  point P0 (0, 0)
  dimension "d247" = 304.8
  dimension "d257" = 152.4
  constraints: 248 end point, 62 parallel, 31 horizontal, 31 perpendicular, 7 point on line, 5 collinear
  measures "d247" distance between parallel lines of L63 L61
  measures "d257" distance between parallel lines of L278 L280
extrude "Extrusion13" add sketch "Sketch3" against normal blind 825.5 contours L174 L75 L168 L244
extrude "Extrusion12" add sketch "Sketch3" against normal blind 762 contours L280 L15 L278 L9
extrude "Extrusion11" add sketch "Sketch3" against normal blind 850.9 contours L24 L180 L274 L5
extrude "Extrusion10" add sketch "Sketch3" against normal blind 800.1 contours L76 L163 L39 L177 | L174 L75 L168 L244 | L161 L263 L147 L39 | L150 L266 L156 L214
extrude "Extrusion9" add sketch "Sketch3" against normal blind 825.5 contours L233 L23 L35 L107 | L104 L284 L98 L282 | L198 L234 L184 L30 | L33 L207 L227 L201 | L225 L93 L35 L21 | L90 L218 L210 L34 | L238 L192 L48 L186 | L120 L66 L142 L272 | L139 L291 L125 L293 | L136 L286 L130 L288
sketch "Sketch5" plane through (-3073.4, 2844.8, 8572.5) normal (0, 0, 1) x (1, 0, 0)
  line L0 (3352.8, -2844.8) -> (5486.4, -2844.8) projected
  line L1 (165.1, -2844.8) -> (3200.4, -2844.8) projected
  line L2 (704.85, -457.2) -> (1371.6, -457.2)
  line L3 (1371.6, -457.2) -> (1371.6, -2057.4)
  line L4 (1371.6, -2057.4) -> (704.85, -2057.4)
  line L5 (704.85, -2057.4) -> (704.85, -457.2)
  line L6 (2228.85, -457.2) -> (2895.6, -457.2)
  line L7 (2895.6, -457.2) -> (2895.6, -2057.4)
  line L8 (2895.6, -2057.4) -> (2228.85, -2057.4)
  line L9 (2228.85, -2057.4) -> (2228.85, -457.2)
  line L10 (3200.4, -2844.8) -> (3200.4, 0) projected
  line L11 (4563.2497, -457.2) -> (5229.9997, -457.2)
  line L12 (5229.9997, -457.2) -> (5229.9997, -2057.4)
  line L13 (5229.9997, -2057.4) -> (4563.2497, -2057.4)
  line L14 (4563.2497, -2057.4) -> (4563.2497, -457.2)
  line L15 (3352.8, 0) -> (3352.8, -2844.8) projected
  line L16 (0, 0) -> (0, -3308.35) projected
  point P0 (3073.4, -2844.8)
  point P1 (1038.225, -2057.4)
  point P2 (2562.225, -2057.4)
  dimension "d268" = 1600.2
  dimension "d270" = 787.4
  dimension "d271" = 666.75
  dimension "d272" = 666.75
  dimension "d274" = 1524
  dimension "d276" = 304.8
  dimension "d277" = 666.75
  dimension "d322" = 5229.9997
  constraints: 24 end point, 6 parallel, 3 collinear, 3 horizontal, 3 perpendicular, 2 midpoint, 1 point on line
  measures "d268" distance between parallel lines of L4 L2
  measures "d270" distance between parallel lines of L1 L4
  measures "d271" distance between parallel lines of L3 L5
  measures "d272" distance between parallel lines of L7 L9
  measures "d274" distance of point (1038.225, -2057.4) point (2562.225, -2057.4)
  measures "d276" distance between parallel lines of L10 L7
  measures "d277" distance between parallel lines of L12 L14
  measures "d322" distance between parallel lines of L16 L12
extrude "Extrusion14" cut sketch "Sketch5" against normal up to surface (165.1 mm away)
sketch "Sketch6" plane through (3073.4, 2844.8, 8572.5) normal (1, 0, 0) x (0, 0, -1)
  line L0 (8712.2, -2844.8) -> (8712.2, 0) projected
  line L1 (5854.7, 0) -> (5854.7, -2844.8) projected
  line L2 (5854.7, -2844.8) -> (8712.2, -2844.8) projected
  line L3 (9563.1, -2844.8) -> (9563.1, 0) projected
  line L4 (8864.6, 0) -> (8864.6, -2844.8) projected
  line L5 (8864.6, -2844.8) -> (9563.1, -2844.8) projected
  line L6 (10287, 0) -> (10287, -2844.8) projected
  line L7 (11188.7, -2844.8) -> (11188.7, 0) projected
  line L8 (10287, -2844.8) -> (11188.7, -2844.8) projected
  line L9 (12922.25, 0) -> (12922.25, -2844.8) projected
  line L10 (14820.9, -2844.8) -> (14820.9, 0) projected
  line L11 (12922.25, -2844.8) -> (14820.9, -2844.8) projected
  line L12 (13074.65, -457.2) -> (13741.4, -457.2)
  line L13 (13741.4, -457.2) -> (13741.4, -2057.4)
  line L14 (13741.4, -2057.4) -> (13074.65, -2057.4)
  line L15 (13074.65, -2057.4) -> (13074.65, -457.2)
  line L16 (6769.1, -457.2) -> (7435.85, -457.2)
  line L17 (7435.85, -457.2) -> (7435.85, -2057.4)
  line L18 (7435.85, -2057.4) -> (6769.1, -2057.4)
  line L19 (6769.1, -2057.4) -> (6769.1, -457.2)
  line L20 (1.5875, 1.5875) -> (17146.5875, 1.5875)
  line L21 (9547.225, -457.2) -> (9547.225, -2057.4)
  line L22 (8880.475, -457.2) -> (9547.225, -457.2)
  line L23 (8880.475, -2057.4) -> (8880.475, -457.2)
  line L24 (9547.225, -2057.4) -> (8880.475, -2057.4)
  line L25 (3.175, 3.175) -> (17148.175, 3.175)
  line L26 (11071.225, -457.2) -> (11071.225, -2057.4)
  line L27 (10404.475, -457.2) -> (11071.225, -457.2)
  line L28 (10404.475, -2057.4) -> (10404.475, -457.2)
  line L29 (11071.225, -2057.4) -> (10404.475, -2057.4)
  point P0 (8572.5, -2844.8)
  point P1 (13408.025, -457.2)
  point P2 (7102.475, -457.2)
  point P3 (8713.7875, 1.5875)
  point P4 (5856.2875, 1.5875)
  point P5 (9564.6875, 1.5875)
  point P6 (8866.1875, 1.5875)
  point P7 (10288.5875, 1.5875)
  point P8 (11190.2875, 1.5875)
  point P9 (12923.8375, 1.5875)
  point P10 (14822.4875, 1.5875)
  point P11 (9213.85, -457.2)
  point P12 (8715.375, 3.175)
  point P13 (5857.875, 3.175)
  point P14 (9566.275, 3.175)
  point P15 (8867.775, 3.175)
  point P16 (10290.175, 3.175)
  point P17 (11191.875, 3.175)
  point P18 (12925.425, 3.175)
  point P19 (14824.075, 3.175)
  point P20 (10737.85, -457.2)
  dimension "d281" = 666.75
  dimension "d284" = 152.4
  dimension "d285" = 787.4
  dimension "d286" = 1600.2
  dimension "d287" = 666.75
  dimension "d288" = 1600.2
  dimension "d289" = 914.4
  dimension "d290" = 787.4
  dimension "d291" = 666.75
  dimension "d292" = 1600.2
  dimension "d293" = 15.875
  dimension "d294" = 787.4
  dimension "d295" = 666.75
  dimension "d296" = 1600.2
  dimension "d297" = 117.475
  dimension "d298" = 787.4
  constraints: 32 end point, 8 parallel, 4 horizontal, 4 midpoint, 4 perpendicular, 6 other
  measures "d281" distance between parallel lines of L13 L15
  measures "d284" distance between parallel lines of L9 L15
  measures "d285" distance between parallel lines of L11 L14
  measures "d286" distance between parallel lines of L14 L12
  measures "d287" distance between parallel lines of L17 L19
  measures "d288" distance between parallel lines of L18 L16
  measures "d289" distance between parallel lines of L1 L19
  measures "d290" distance between parallel lines of L2 L18
  measures "d291" distance between parallel lines of L21 L23
  measures "d292" distance between parallel lines of L24 L22
  measures "d293" distance between parallel lines of L3 L21
  measures "d294" distance between parallel lines of L5 L24
  measures "d295" distance between parallel lines of L26 L28
  measures "d296" distance between parallel lines of L29 L27
  measures "d297" distance between parallel lines of L7 L26
  measures "d298" distance between parallel lines of L8 L29
extrude "Extrusion15" cut sketch "Sketch6" against normal up to surface (165.1 mm away)
sketch "Sketch7" plane through (3073.4, 2844.8, -8572.5) normal (0, 0, -1) x (-1, 0, 0)
  line L0 (6146.8, -3308.35) -> (6146.8, 0) projected
  line L1 (2552.7, -2844.8) -> (5981.7, -2844.8) projected
  line L2 (4695.825, -457.2) -> (5362.575, -457.2)
  line L3 (5362.575, -457.2) -> (5362.575, -2057.4)
  line L4 (5362.575, -2057.4) -> (4695.825, -2057.4)
  line L5 (4695.825, -2057.4) -> (4695.825, -457.2)
  point P0 (3073.4, -2844.8)
  point P1 (5029.2, -2057.4)
  dimension "d301" = 1117.6
  dimension "d302" = 787.4
  dimension "d303" = 1600.2
  dimension "d304" = 666.75
  constraints: 8 end point, 2 parallel, 1 horizontal, 1 midpoint, 1 perpendicular
  measures "d301" distance from line of L0 point (5029.2, -2057.4)
  measures "d302" distance between parallel lines of L1 L4
  measures "d303" distance between parallel lines of L2 L4
  measures "d304" distance between parallel lines of L3 L5
extrude "Extrusion16" cut sketch "Sketch7" against normal up to surface (165.1 mm away)
sketch "Sketch8" plane through (-3073.4, 2844.8, -8572.5) normal (-1, 0, 0) x (0, 0, 1)
  line L0 (6972.3, -2844.8) -> (6972.3, 0) projected
  line L1 (2324.1, 0) -> (2324.1, -2844.8) projected
  line L2 (2324.1, -2844.8) -> (6972.3, -2844.8) projected
  line L3 (2628.9, -457.2) -> (3295.65, -457.2)
  line L4 (3295.65, -457.2) -> (3295.65, -2057.4)
  line L5 (3295.65, -2057.4) -> (2628.9, -2057.4)
  line L6 (2628.9, -2057.4) -> (2628.9, -457.2)
  line L7 (5594.35, -457.2) -> (6261.1, -457.2)
  line L8 (6261.1, -457.2) -> (6261.1, -2057.4)
  line L9 (6261.1, -2057.4) -> (5594.35, -2057.4)
  line L10 (5594.35, -2057.4) -> (5594.35, -457.2)
  line L11 (9283.7, -641.35) -> (10071.1, -641.35)
  line L12 (10071.1, -641.35) -> (10071.1, -1987.55)
  line L13 (10071.1, -1987.55) -> (9283.7, -1987.55)
  line L14 (9283.7, -1987.55) -> (9283.7, -641.35)
  line L15 (11195.05, -641.35) -> (11982.45, -641.35)
  line L16 (11982.45, -641.35) -> (11982.45, -1987.55)
  line L17 (11982.45, -1987.55) -> (11195.05, -1987.55)
  line L18 (11195.05, -1987.55) -> (11195.05, -641.35)
  line L19 (8432.8, 0) -> (8432.8, -2844.8) projected
  line L20 (8432.8, -2844.8) -> (12763.5, -2844.8) projected
  line L21 (17145, 0) -> (17145, -3308.35) projected
  line L22 (0, 0) -> (17145, 0) projected
  line L23 (0, -3308.35) -> (0, 0) projected
  line L24 (17145, -3308.35) -> (0, -3308.35) projected
  line L25 (12763.5, -2844.8) -> (12763.5, 0) projected
  line L26 (2628.9, -457.2) -> (3295.65, -457.2)
  line L27 (3295.65, -457.2) -> (3295.65, -2057.4)
  line L28 (3295.65, -2057.4) -> (2628.9, -2057.4)
  line L29 (2628.9, -2057.4) -> (2628.9, -457.2)
  line L30 (5594.35, -2057.4) -> (6261.1, -2057.4)
  line L31 (6261.1, -2057.4) -> (6261.1, -457.2)
  line L32 (6261.1, -457.2) -> (5594.35, -457.2)
  line L33 (5594.35, -457.2) -> (5594.35, -2057.4)
  line L34 (9283.7, -641.35) -> (10071.1, -641.35)
  line L35 (10071.1, -641.35) -> (10071.1, -1987.55)
  line L36 (10071.1, -1987.55) -> (9283.7, -1987.55)
  line L37 (9283.7, -1987.55) -> (9283.7, -641.35)
  line L38 (11195.05, -1987.55) -> (11982.45, -1987.55)
  line L39 (11982.45, -1987.55) -> (11982.45, -641.35)
  line L40 (11982.45, -641.35) -> (11195.05, -641.35)
  line L41 (11195.05, -641.35) -> (11195.05, -1987.55)
  point P0 (8572.5, -2844.8)
  point P1 (9677.4, -1987.55)
  dimension "d307" = 304.8
  dimension "d308" = 711.2
  dimension "d309" = 1244.6
  dimension "d311" = 781.05
  dimension "d312" = 857.25
  dimension "d313" = 1346.2
  dimension "d314" = 787.4
  dimension "d315" = 787.4
  dimension "d316" = 787.4
  dimension "d317" = 666.75
  dimension "d318" = 1600.2
  dimension "d319" = 666.75
  constraints: 64 end point, 16 parallel, 8 horizontal, 8 perpendicular, 4 collinear, 1 midpoint
  measures "d307" distance between parallel lines of L1 L6
  measures "d308" distance between parallel lines of L0 L8
  measures "d309" distance from line of L19 point (9677.4, -1987.55)
  measures "d311" distance between parallel lines of L25 L16
  measures "d312" distance between parallel lines of L20 L13
  measures "d313" distance from line of point (9677.4, -1987.55) L11
  measures "d314" distance between parallel lines of L12 L14
  measures "d315" distance between parallel lines of L16 L18
  measures "d316" distance between parallel lines of L2 L5
  measures "d317" distance between parallel lines of L6 L4
  measures "d318" distance between parallel lines of L5 L3
  measures "d319" distance between parallel lines of L8 L10
extrude "Extrusion17" cut sketch "Sketch8" against normal up to surface (165.1 mm away) contours L3 L4 L5 L6 | L7 L8 L9 L10 | L11 L12 L13 L14 | L15 L16 L17 L18
sketch "Sketch4" plane through (0, 2844.8, 0) normal (0, 1, 0) x (1, 0, 0)
  line L0 (1739.9, -3841.75) -> (1739.9, -2832.1) projected
  line L1 (2908.3, -2832.1) -> (1739.9, -2832.1) projected
  line L2 (2908.3, -2832.1) -> (2908.3, -4762.5) projected
  line L3 (1993.9, -4762.5) -> (2908.3, -4762.5) projected
  line L4 (1993.9, -3841.75) -> (1993.9, -4762.5) projected
  line L5 (1739.9, -3841.75) -> (1993.9, -3841.75) projected
  point P0 (0, 0)
body "Solid1"
